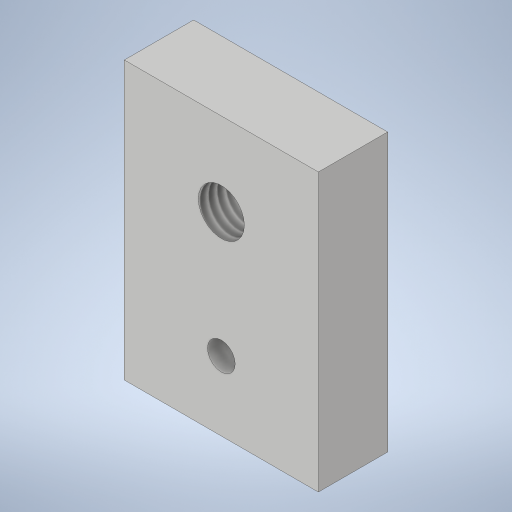
# Autodesk Inventor part: Guia sujecion centellador
Saved by Autodesk Inventor 2024.2 (Build 282272000, 272)
## iProperties
Created: 2025-06-17
Part Number: Guia sujecion centellador
Material: Genérico
Document SubType Name: Modeling
Designer: jd.castellanosq
Density: 1 g/cm^3
Appearance: Valor por defecto
Author: jd.castellanosq
Autodesk Inventor part; units mm, degrees
ref_plane "YZ Plane" through (0, 0, 0) normal (1, 0, 0) x (0, 1, 0)
ref_plane "XZ Plane" through (0, 0, 0) normal (0, 1, 0) x (-1, 0, 0)
ref_plane "XY Plane" through (0, 0, 0) normal (0, 0, 1) x (1, 0, 0)
sketch "Boceto1" plane through (0, 0, 0) normal (0, 1, 0) x (-1, 0, 0)
  line L0 (14, -5) -> (-14, -5)
  line L1 (-14, -5) -> (-14, 5)
  line L2 (-14, 5) -> (14, 5)
  line L3 (14, 5) -> (14, -5)
  point P0 (0, 0)
  point P1 (0, -5)
  point P2 (-14, 0)
  dimension "d0" = 28
  dimension "d1" = 10
  constraints: 8 end point, 2 midpoint, 2 parallel, 1 horizontal, 1 horizontal alignment, 1 perpendicular, 1 vertical alignment
  measures "d0" distance of L0.start L0.end
  measures "d1" distance of L0.end L1.end
extrude "Extrusión1" add sketch "Boceto1" along normal blind 40
sketch "Boceto2" plane through (0, 0, 0) normal (0, -1, 0) x (1, 0, 0)
  point P0 (0, 0)
  point P1 (6, 0)
  point P2 (-6, 0)
  dimension "d19" = 12
  dimension "d20" = 6
  constraints: 2 horizontal alignment
  measures "d19" distance of point (-6, 0) point (6, 0)
  measures "d20" distance of point (-6, 0) point (0, 0)
hole "Agujero1" at (6, 0, 0) at (-6, 0, 0) direction (0, 1, 0) diameter 3.242 depth 11.8 tip angle 118 thread size "M4x0.7" class "6H" standard "ANSI Metric M Profile"
sketch "Boceto3" plane through (-14, 0, 5) normal (0, 0, 1) x (1, 0, 0)
  line L0 (0, 0) -> (28, 0) projected
  point P0 (14, 0)
  point P1 (14, 28)
  point P2 (14, 0)
  dimension "d11" = 28
  constraints: 1 midpoint, 1 vertical alignment
  measures "d11" distance from line of point (14, 28) L0
hole "Agujero2" at (0, 28, 5) direction (0, 0, -1) diameter 6.647 end through all thread size "M8x1.25" class "6H" standard "ANSI Metric M Profile"
sketch "Boceto4" plane through (-14, 0, 5) normal (0, 0, 1) x (1, 0, 0)
  circle A0 centre (14, 10) radius 2
  line L0 (0, 0) -> (28, 0) projected
  point P0 (14, 0)
  point P1 (14, 0)
  dimension "d21" = 4
  dimension "d22" = 10
  constraints: 1 centre point, 1 midpoint, 1 vertical alignment
  measures "d21" diameter of A0
  measures "d22" distance from line of A0.centre L0
extrude "Extrusión2" cut sketch "Boceto4" against normal blind 10
equation "\"d20\" = 0.5 * d19"
